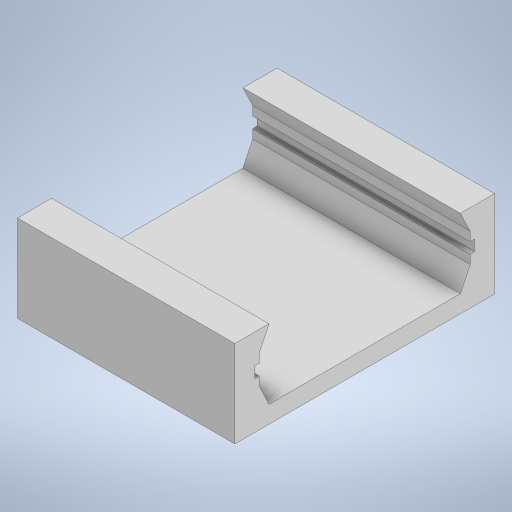
# Autodesk Inventor part: RaspberryPi Camera Slotted Mount
Saved by Autodesk Inventor 2023 (Build 270158000, 158)
## iProperties
Created: 2023-04-05
Part Number: RaspberryPi Camera Slotted Mount
Material: Generic
Document SubType Name: Modeling
Designer: Administrator
Density: 1 g/cm^3
Appearance: Default
Author: Administrator
Autodesk Inventor part; units mm, degrees
ref_plane "YZ Plane" through (0, 0, 0) normal (1, 0, 0) x (0, 1, 0)
ref_plane "XZ Plane" through (0, 0, 0) normal (0, 1, 0) x (-1, 0, 0)
ref_plane "XY Plane" through (0, 0, 0) normal (0, 0, 1) x (1, 0, 0)
sketch "Sketch1" plane through (0, 0, 0) normal (1, 0, 0) x (0, 1, 0)
  line L0 (0, 0) -> (1.25, 0)
  line L1 (1.25, 0) -> (1.25, -25.25)
  line L2 (1.25, -25.25) -> (0, -25.25)
  line L3 (0, -25.25) -> (0, 0)
  line L4 (4.625, -1.625) -> (0.625, 0.3009)
  line L5 (0.625, 0.3009) -> (-3.375, -1.625)
  line L6 (-3.375, -23.625) -> (0.625, -25.5509)
  line L7 (0.625, -25.5509) -> (4.625, -23.625)
  line L8 (4.625, 2.3009) -> (-3.375, 2.3009)
  line L9 (-3.375, 2.3009) -> (-3.375, -27.5509)
  line L10 (-3.375, -27.5509) -> (4.625, -27.5509)
  line L11 (4.625, -27.5509) -> (4.625, 2.3009)
  line L12 (-3.375, 2.3009) -> (-5.375, 2.3009)
  line L13 (-5.375, 2.3009) -> (-5.375, -27.5509)
  line L14 (-5.375, -27.5509) -> (-3.375, -27.5509)
  line L15 (-3.375, -27.5509) -> (-3.375, 2.3009)
  line L16 (-1.0385, -0.5) -> (2.2885, -0.5)
  line L17 (-1.0385, -24.75) -> (2.2885, -24.75)
  point P0 (0, -24.75)
  point P1 (0, -0.5)
  point P2 (1.25, -0.5)
  point P3 (1.25, -24.75)
  dimension "d0" = 1.25
  dimension "d1" = 25.25
  dimension "d2" = 0.625
  dimension "d3" = 2
  dimension "d4" = 2
  dimension "d5" = 8
  dimension "d6" = 22
  dimension "d7" = 2
  dimension "d8" = 0.5
  dimension "d9" = 0.5
  constraints: 36 end point, 12 point on line, 8 parallel, 5 horizontal, 3 perpendicular, 1 equal length
  measures "d0" distance of L1.end L2.end
  measures "d1" distance of L0.end L1.end
  measures "d2" horizontal distance of L2.end L6.end
  measures "d3" distance from line of L8 L4.end
  measures "d4" distance from line of L6.end L10
  measures "d5" distance of L9.end L10.end
  measures "d6" distance of L7.end L4.start
  measures "d7" distance of L9.end L13.end
  measures "d8" distance between parallel lines of L16 L0
  measures "d9" distance between parallel lines of L2 L17
extrude "Extrusion1" add sketch "Sketch1" along normal blind 25 contours L5 L4 L0 | L5 L9 L8 L11 L4 | L3 L16 L5 | L4 L16 L1 | L3 L6 L17 | L9 L14 L13 L12 | L17 L7 L1 | L6 L7 L11 L10 L9 | L2 L7 L6
equation "\"d2\" = 0.5 * d0"
body "Solid1"
